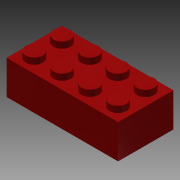
# Autodesk Inventor part: Lego_Brick
Saved by Autodesk Inventor 2015 (Build 190159000, 159)
## iProperties
Created: 2013-05-23
Material: PC/ABS Plastic
Document SubType Name: Modeling
Density: 0.357273 g/cm^3
Appearance: Smooth - White
Autodesk Inventor part; units mm, degrees
sketch "Sketch1" plane through (0, 0, 0) normal (0, 1, 0) x (-1, 0, 0)
  line L0 (0, 0) -> (31.75, 0)
  line L1 (31.75, 0) -> (31.75, 15.748)
  line L2 (31.75, 15.748) -> (0, 15.748)
  line L3 (0, 15.748) -> (0, 0)
  dimension "d0" = 31.75
  dimension "d2" = 15.748
  constraints: 8 end point, 2 parallel, 1 horizontal, 1 perpendicular
  measures "d0" distance of L1.end L2.end
  measures "d2" distance of L0.end L1.end
extrude "Extrusion1" add sketch "Sketch1" along normal blind 9.652
ref_plane "Work Plane1" through (0, 9.652, 0) normal (0, 1, 0) x (1, 0, 0)
sketch "Sketch2" plane through (0, 9.652, 0) normal (0, 1, 0) x (1, 0, 0)
  circle A0 centre (-3.9751, -3.937) radius 2.413
  circle A1 centre (-11.9126, -3.937) radius 2.413
  circle A2 centre (-19.8501, -3.937) radius 2.413
  circle A3 centre (-27.7876, -3.937) radius 2.413
  circle A4 centre (-3.9751, -11.811) radius 2.413
  circle A5 centre (-11.9126, -11.811) radius 2.413
  circle A6 centre (-19.8501, -11.811) radius 2.413
  circle A7 centre (-27.7876, -11.811) radius 2.413
  point P0 (0, 0)
  dimension "d17" = 4.826
  dimension "d19" = 4.826
  dimension "d21" = 4.826
  dimension "d23" = 4.826
  dimension "d25" = 4.826
  dimension "d29" = 4.826
  dimension "d30" = 4.826
  dimension "d31" = 4.826
  constraints: 8 centre point
  measures "d17" diameter of A0
  measures "d19" diameter of A1
  measures "d21" diameter of A2
  measures "d23" diameter of A3
  measures "d25" diameter of A4
  measures "d29" diameter of A5
  measures "d30" diameter of A6
  measures "d31" diameter of A7
extrude "Extrusion2" add sketch "Sketch2" along normal blind 1.778
ref_plane "Work Plane2" through (0, 0, 0) normal (0, -1, 0) x (1, 0, 0)
sketch "Sketch3" plane through (0, 0, 0) normal (0, -1, 0) x (1, 0, 0)
  line L0 (-1.27, 1.27) -> (-30.48, 1.27)
  line L1 (-30.48, 1.27) -> (-30.48, 14.478)
  line L2 (-1.27, 14.478) -> (-1.27, 1.27)
  line L3 (-28.0988, 1.27) -> (-27.4638, 1.27)
  line L4 (-27.4638, 1.27) -> (-27.4638, 1.524)
  line L5 (-27.4638, 1.524) -> (-28.0988, 1.524)
  line L6 (-28.0988, 1.524) -> (-28.0988, 1.27)
  line L7 (-28.0988, 1.27) -> (-27.4638, 1.524) construction
  line L8 (-27.4638, 1.27) -> (-28.0988, 1.524) construction
  line L9 (-20.1612, 1.524) -> (-19.5262, 1.524)
  line L10 (-19.5262, 1.524) -> (-19.5262, 1.27)
  line L11 (-19.5262, 1.27) -> (-20.1612, 1.27)
  line L12 (-20.1612, 1.27) -> (-20.1612, 1.524)
  line L13 (-20.1612, 1.524) -> (-19.5262, 1.27) construction
  line L14 (-19.5262, 1.524) -> (-20.1612, 1.27) construction
  line L15 (-12.2237, 1.524) -> (-11.5887, 1.524)
  line L16 (-11.5887, 1.524) -> (-11.5887, 1.27)
  line L17 (-11.5887, 1.27) -> (-12.2237, 1.27)
  line L18 (-12.2237, 1.27) -> (-12.2237, 1.524)
  line L19 (-12.2237, 1.524) -> (-11.5887, 1.27) construction
  line L20 (-11.5887, 1.524) -> (-12.2237, 1.27) construction
  line L21 (-4.2862, 1.524) -> (-3.6512, 1.524)
  line L22 (-3.6512, 1.524) -> (-3.6512, 1.27)
  line L23 (-3.6512, 1.27) -> (-4.2862, 1.27)
  line L24 (-4.2862, 1.27) -> (-4.2862, 1.524)
  line L25 (-4.2862, 1.524) -> (-3.6512, 1.27) construction
  line L26 (-3.6512, 1.524) -> (-4.2862, 1.27) construction
  line L27 (-1.27, 14.478) -> (-30.48, 14.478)
  line L28 (-28.0988, 14.478) -> (-27.4638, 14.478)
  line L29 (-27.4638, 14.478) -> (-27.4638, 14.224)
  line L30 (-27.4638, 14.224) -> (-28.0988, 14.224)
  line L31 (-28.0988, 14.224) -> (-28.0988, 14.478)
  line L32 (-20.1612, 14.224) -> (-19.5262, 14.224)
  line L33 (-19.5262, 14.224) -> (-19.5262, 14.478)
  line L34 (-19.5262, 14.478) -> (-20.1612, 14.478)
  line L35 (-20.1612, 14.478) -> (-20.1612, 14.224)
  line L36 (-12.2237, 14.224) -> (-11.5887, 14.224)
  line L37 (-11.5887, 14.224) -> (-11.5887, 14.478)
  line L38 (-11.5887, 14.478) -> (-12.2237, 14.478)
  line L39 (-12.2237, 14.478) -> (-12.2237, 14.224)
  line L40 (-4.2862, 14.224) -> (-3.6512, 14.224)
  line L41 (-3.6512, 14.224) -> (-3.6512, 14.478)
  line L42 (-3.6512, 14.478) -> (-4.2862, 14.478)
  line L43 (-4.2862, 14.478) -> (-4.2862, 14.224)
  line L44 (-1.27, 1.27) -> (-1.27, 5.207)
  line L45 (-30.48, 12.1285) -> (-30.48, 11.4935)
  line L46 (-30.48, 11.4935) -> (-30.226, 11.4935)
  line L47 (-30.226, 11.4935) -> (-30.226, 12.1285)
  line L48 (-30.226, 12.1285) -> (-30.48, 12.1285)
  line L49 (-30.48, 12.1285) -> (-30.226, 11.4935) construction
  line L50 (-30.48, 11.4935) -> (-30.226, 12.1285) construction
  line L51 (-30.48, 5.5245) -> (-30.48, 4.8895)
  line L52 (-30.48, 4.8895) -> (-30.226, 4.8895)
  line L53 (-30.226, 4.8895) -> (-30.226, 5.5245)
  line L54 (-30.226, 5.5245) -> (-30.48, 5.5245)
  line L55 (-30.48, 5.5245) -> (-30.226, 4.8895) construction
  line L56 (-30.48, 4.8895) -> (-30.226, 5.5245) construction
  line L57 (-1.27, 12.1285) -> (-1.27, 11.4935)
  line L58 (-1.27, 11.4935) -> (-1.524, 11.4935)
  line L59 (-1.524, 11.4935) -> (-1.524, 12.1285)
  line L60 (-1.524, 12.1285) -> (-1.27, 12.1285)
  line L61 (-1.27, 12.1285) -> (-1.524, 11.4935) construction
  line L62 (-1.27, 11.4935) -> (-1.524, 12.1285) construction
  line L63 (-1.27, 5.5245) -> (-1.27, 4.8895)
  line L64 (-1.27, 4.8895) -> (-1.524, 4.8895)
  line L65 (-1.524, 4.8895) -> (-1.524, 5.5245)
  line L66 (-1.524, 5.5245) -> (-1.27, 5.5245)
  line L67 (-1.27, 5.5245) -> (-1.524, 4.8895) construction
  line L68 (-1.27, 4.8895) -> (-1.524, 5.5245) construction
  point P0 (0, 0)
  dimension "d48" = 0.635
  dimension "d49" = 0.254
  dimension "d50" = 0.635
  dimension "d51" = 0.254
  dimension "d52" = 0.635
  dimension "d53" = 0.254
  dimension "d54" = 0.635
  dimension "d55" = 0.254
  dimension "d58" = 3.937
  dimension "d65" = 0.635
  dimension "d66" = 0.254
  dimension "d67" = 0.635
  dimension "d68" = 0.254
  constraints: 138 end point, 13 parallel, 7 perpendicular, 5 horizontal, 5 point on line, 2 collinear
  measures "d48" distance of L5.end L4.end
  measures "d49" distance of L3.end L4.end
  measures "d50" distance of L10.end L11.end
  measures "d51" distance of L9.end L10.end
  measures "d52" distance of L16.end L17.end
  measures "d53" distance of L15.end L16.end
  measures "d54" distance of L22.end L23.end
  measures "d55" distance of L21.end L22.end
  measures "d58" distance of L0.start L44.end
  measures "d65" distance of L45.start L45.end
  measures "d66" distance of L46.end L45.end
  measures "d67" distance of L51.start L51.end
  measures "d68" distance of L52.end L51.end
extrude "Extrusion3" cut sketch "Sketch3" against normal blind 8.382 contours L0 L22 L21 L24 L16 L15 L18 L10 L9 L12 L4 L5 L6 L1 L52 L53 L54 L46 L47 L48 L27 L31 L30 L29 L35 L32 L33 L39 L36 L37 L43 L40 L41 L2 L60 L59 L58 L66 L65 L64
ref_plane "Work Plane3" through (0, 8.382, 0) normal (0, -1, 0) x (1, 0, 0)
sketch "Sketch4" plane through (0, 8.382, 0) normal (0, -1, 0) x (1, 0, 0)
  circle A0 centre (-23.8125, 7.874) radius 3.302
  circle A1 centre (-15.875, 7.874) radius 3.302
  circle A2 centre (-7.9375, 7.874) radius 3.302
  circle A3 centre (-23.8125, 7.874) radius 2.8575
  circle A4 centre (-15.875, 7.874) radius 2.8575
  circle A5 centre (-7.9375, 7.874) radius 2.8575
  point P0 (0, 0)
  dimension "d78" = 6.604
  dimension "d79" = 6.604
  dimension "d80" = 6.604
  dimension "d81" = 5.715
  dimension "d82" = 5.715
  dimension "d83" = 5.715
  constraints: 6 centre point, 3 coincident
  measures "d78" diameter of A0
  measures "d79" diameter of A1
  measures "d80" diameter of A2
  measures "d81" diameter of A3
  measures "d82" diameter of A4
  measures "d83" diameter of A5
extrude "Extrusion4" add sketch "Sketch4" along normal blind 8.382
sketch "Sketch5" plane through (0, 8.382, 0) normal (0, -1, 0) x (1, 0, 0)
  line L0 (-15.4305, 4.572) -> (-15.4305, 1.27)
  line L1 (-15.4305, 1.27) -> (-16.3195, 1.27)
  line L2 (-16.3195, 1.27) -> (-16.3195, 4.572)
  line L3 (-16.3195, 4.572) -> (-15.4305, 1.27) construction
  line L4 (-15.4305, 4.572) -> (-16.3195, 1.27) construction
  line L5 (-16.3195, 4.572) -> (-16.3195, 4.6021)
  line L6 (-15.4305, 4.572) -> (-15.4305, 4.6021)
  line L7 (-15.4305, 11.176) -> (-15.4305, 14.478)
  line L8 (-15.4305, 14.478) -> (-16.3195, 14.478)
  line L9 (-16.3195, 14.478) -> (-16.3195, 11.176)
  line L10 (-16.3195, 11.176) -> (-15.4305, 14.478) construction
  line L11 (-15.4305, 11.176) -> (-16.3195, 14.478) construction
  line L12 (-16.3195, 11.176) -> (-16.3195, 11.1459)
  line L13 (-15.4305, 11.176) -> (-15.4305, 11.1459)
  arc A0 (-15.4305, 11.1459) -> (-16.3195, 11.1459) centre (-15.875, 7.874) ccw
  arc A1 (-16.3195, 4.6021) -> (-15.4305, 4.6021) centre (-15.875, 7.874) ccw
  point P0 (0, 0)
  point P1 (-15.875, 2.921)
  point P2 (-15.875, 12.827)
  dimension "d92" = 0.889
  dimension "d93" = 0.889
  constraints: 28 end point, 4 midpoint, 4 parallel, 4 point on circle, 2 centre point, 2 collinear
  measures "d92" distance of L0.end L1.end
  measures "d93" distance of L8.end L7.end
extrude "Extrusion5" add sketch "Sketch5" along normal blind 6.8499
fillet "Fillet2" radius 0.127 3 edges at (-10.795, 0, 7.874) (-18.7325, 0, 7.874) (-26.67, 0, 7.874)
ref_plane "Work Plane4" through (-19.5262, 0, 1.27) normal (0, 0, 1) x (1, 0, 0)
sketch "Sketch6" plane through (-19.5262, 0, 1.27) normal (0, 0, 1) x (1, 0, 0)
  arc A0 (3.2067, 1.5321) -> (4.0957, 1.5321) centre (3.6512, 1.778) ccw
  line L0 (4.0957, 1.5321) -> (3.2067, 1.5321)
  point P0 (19.5262, 0)
  dimension "d104" = 0.889
  dimension "d108" = 0.508
  constraints: 2 end point, 2 point on circle, 1 centre point, 1 horizontal
  measures "d104" distance of L0.start L0.end
  measures "d108" radius of A0
extrude "Extrusion6" add sketch "Sketch6" along normal up to next
ref_plane "Work Plane5" through (-12.2237, 0, 14.478) normal (0, 0, -1) x (-1, 0, 0)
sketch "Sketch7" plane through (-12.2237, 0, 14.478) normal (0, 0, -1) x (-1, 0, 0)
  arc A0 (3.2067, 1.5321) -> (4.0957, 1.5321) centre (3.6512, 1.778) ccw
  line L0 (4.0957, 1.5321) -> (3.2067, 1.5321)
  point P0 (-12.2237, 0)
  dimension "d111" = 0.889
  dimension "d112" = 0.508
  constraints: 2 end point, 2 point on circle, 1 centre point, 1 horizontal
  measures "d111" distance of L0.start L0.end
  measures "d112" radius of A0
extrude "Extrusion7" add sketch "Sketch7" along normal up to next
body "Solid1"
